Autodesk Fusion 360 part; units mm, degrees
(part 2 of 5)
sketch "Sketch20" plane through (0, 0, 3.3) normal (0, 0, 1) x (-1, 0, 0)
  arc A0 (-66.5616, 3.5945) -> (-66.8099, 2.6679) centre (-55, 0) ccw
  arc A1 (-67.9306, 1.8988) -> (-66.8099, 2.6679) centre (-67.7853, 2.8882) ccw
  line L0 (-67.9306, 1.8988) -> (-68.9458, 2.0479)
  spline S0 degree 5 poles (-68.9458, 2.0479) (-68.9559, 2.0494) (-68.9759, 2.052) (-69.0061, 2.055) (-69.0465, 2.0571) (-69.0972, 2.0572) (-69.1481, 2.0556) (-69.199, 2.0528) (-69.2501, 2.0495) (-69.3011, 2.0457) (-69.3522, 2.0415) (-69.4034, 2.0367) (-69.4546, 2.0311) (-69.5058, 2.0247) (-69.5571, 2.0173) (-69.6084, 2.0092) (-69.6597, 2.0003) (-69.7111, 1.9908) (-69.7624, 1.9808) (-69.8137, 1.9703) (-69.8651, 1.9594) (-69.9164, 1.9479) (-69.9678, 1.9358) (-70.0191, 1.9232) (-70.0705, 1.91) (-70.1218, 1.8963) (-70.1731, 1.882) (-70.2244, 1.8673) (-70.2757, 1.8521) (-70.3269, 1.8365) (-70.3781, 1.8204) (-70.4293, 1.8038) (-70.4805, 1.7868) (-70.5316, 1.7693) (-70.5827, 1.7513) (-70.6338, 1.7329) (-70.6848, 1.7141) (-70.7358, 1.6948) (-70.7868, 1.6751) (-70.8377, 1.655) (-70.8886, 1.6345) (-70.9394, 1.6136) (-70.9902, 1.5922) (-71.0409, 1.5705) (-71.0916, 1.5483) (-71.1422, 1.5258) (-71.1928, 1.5028) (-71.2433, 1.4794) (-71.2937, 1.4557) (-71.3441, 1.4316) (-71.3944, 1.4071) (-71.4447, 1.3822) (-71.4949, 1.3569) (-71.545, 1.3313) (-71.5951, 1.3053) (-71.6451, 1.2789) (-71.695, 1.2521) (-71.7448, 1.225) (-71.7946, 1.1975) (-71.8443, 1.1697) (-71.8939, 1.1415) (-71.9435, 1.1129) (-71.9929, 1.084) (-72.0423, 1.0548) (-72.0916, 1.0251) (-72.1408, 0.9952) (-72.1899, 0.9649) (-72.239, 0.9343) (-72.2879, 0.9033) (-72.3368, 0.8719) (-72.3856, 0.8403) (-72.4245, 0.8147) (-72.4537, 0.7953) (-72.4731, 0.7824) (-72.4828, 0.7759) knots 0 0 0 0 0 0 0.01428571 0.02857143 0.04285714 0.05714286 0.07142857 0.08571429 0.1 0.11428571 0.12857143 0.14285714 0.15714286 0.17142857 0.18571429 0.2 0.21428571 0.22857143 0.24285714 0.25714286 0.27142857 0.28571429 0.3 0.31428571 0.32857143 0.34285714 0.35714286 0.37142857 0.38571429 0.4 0.41428571 0.42857143 0.44285714 0.45714286 0.47142857 0.48571429 0.5 0.51428571 0.52857143 0.54285714 0.55714286 0.57142857 0.58571429 0.6 0.61428571 0.62857143 0.64285714 0.65714286 0.67142857 0.68571429 0.7 0.71428571 0.72857143 0.74285714 0.75714286 0.77142857 0.78571429 0.8 0.81428571 0.82857143 0.84285714 0.85714286 0.87142857 0.88571429 0.9 0.91428571 0.92857143 0.94285714 0.95714286 0.97142857 0.98571429 1 1 1 1 1 1
  arc A2 (-72.4828, 0.7759) -> (-72.4828, -0.7759) centre (-55, 0) ccw
  spline S1 degree 5 poles (-72.4828, -0.7759) (-72.4731, -0.7824) (-72.4537, -0.7953) (-72.4245, -0.8147) (-72.3856, -0.8403) (-72.3368, -0.8719) (-72.2879, -0.9033) (-72.239, -0.9343) (-72.1899, -0.9649) (-72.1408, -0.9952) (-72.0916, -1.0251) (-72.0423, -1.0548) (-71.9929, -1.084) (-71.9435, -1.1129) (-71.8939, -1.1415) (-71.8443, -1.1697) (-71.7946, -1.1975) (-71.7448, -1.225) (-71.695, -1.2521) (-71.6451, -1.2789) (-71.5951, -1.3053) (-71.545, -1.3313) (-71.4949, -1.3569) (-71.4447, -1.3822) (-71.3944, -1.4071) (-71.3441, -1.4316) (-71.2937, -1.4557) (-71.2433, -1.4794) (-71.1928, -1.5028) (-71.1422, -1.5258) (-71.0916, -1.5483) (-71.0409, -1.5705) (-70.9902, -1.5922) (-70.9394, -1.6136) (-70.8886, -1.6345) (-70.8377, -1.655) (-70.7868, -1.6751) (-70.7358, -1.6948) (-70.6848, -1.7141) (-70.6338, -1.7329) (-70.5827, -1.7513) (-70.5316, -1.7693) (-70.4805, -1.7868) (-70.4293, -1.8038) (-70.3781, -1.8204) (-70.3269, -1.8365) (-70.2757, -1.8521) (-70.2244, -1.8673) (-70.1731, -1.882) (-70.1218, -1.8963) (-70.0705, -1.91) (-70.0191, -1.9232) (-69.9678, -1.9358) (-69.9164, -1.9479) (-69.8651, -1.9594) (-69.8137, -1.9703) (-69.7624, -1.9808) (-69.7111, -1.9908) (-69.6597, -2.0003) (-69.6084, -2.0092) (-69.5571, -2.0173) (-69.5058, -2.0247) (-69.4546, -2.0311) (-69.4034, -2.0367) (-69.3522, -2.0415) (-69.3011, -2.0457) (-69.2501, -2.0495) (-69.199, -2.0528) (-69.1481, -2.0556) (-69.0972, -2.0572) (-69.0465, -2.0571) (-69.0061, -2.055) (-68.9759, -2.052) (-68.9559, -2.0494) (-68.9458, -2.0479) knots -1 -1 -1 -1 -1 -1 -0.98571429 -0.97142857 -0.95714286 -0.94285714 -0.92857143 -0.91428571 -0.9 -0.88571429 -0.87142857 -0.85714286 -0.84285714 -0.82857143 -0.81428571 -0.8 -0.78571429 -0.77142857 -0.75714286 -0.74285714 -0.72857143 -0.71428571 -0.7 -0.68571429 -0.67142857 -0.65714286 -0.64285714 -0.62857143 -0.61428571 -0.6 -0.58571429 -0.57142857 -0.55714286 -0.54285714 -0.52857143 -0.51428571 -0.5 -0.48571429 -0.47142857 -0.45714286 -0.44285714 -0.42857143 -0.41428571 -0.4 -0.38571429 -0.37142857 -0.35714286 -0.34285714 -0.32857143 -0.31428571 -0.3 -0.28571429 -0.27142857 -0.25714286 -0.24285714 -0.22857143 -0.21428571 -0.2 -0.18571429 -0.17142857 -0.15714286 -0.14285714 -0.12857143 -0.11428571 -0.1 -0.08571429 -0.07142857 -0.05714286 -0.04285714 -0.02857143 -0.01428571 0 0 0 0 0 0
  line L1 (-68.9458, -2.0479) -> (-67.9306, -1.8988)
  arc A3 (-66.8099, -2.6679) -> (-67.9306, -1.8988) centre (-67.7853, -2.8882) ccw
  arc A4 (-66.8099, -2.6679) -> (-66.5616, -3.5945) centre (-55, 0) ccw
  arc A5 (-67.1477, -4.8209) -> (-66.5616, -3.5945) centre (-67.5165, -3.8914) ccw
  line L2 (-67.1477, -4.8209) -> (-68.1014, -5.1994)
  spline S2 degree 5 poles (-68.1014, -5.1994) (-68.1108, -5.2031) (-68.1295, -5.2109) (-68.1571, -5.2234) (-68.1932, -5.2418) (-68.2372, -5.267) (-68.2804, -5.2939) (-68.3231, -5.3217) (-68.3657, -5.3501) (-68.408, -5.3789) (-68.4502, -5.4081) (-68.4921, -5.4379) (-68.5336, -5.4683) (-68.5747, -5.4995) (-68.6155, -5.5315) (-68.6558, -5.5642) (-68.6958, -5.5976) (-68.7355, -5.6314) (-68.775, -5.6658) (-68.8143, -5.7005) (-68.8532, -5.7357) (-68.8919, -5.7713) (-68.9304, -5.8074) (-68.9685, -5.844) (-69.0064, -5.8811) (-69.044, -5.9187) (-69.0813, -5.9566) (-69.1184, -5.995) (-69.1552, -6.0338) (-69.1917, -6.073) (-69.228, -6.1126) (-69.2641, -6.1525) (-69.2999, -6.1929) (-69.3354, -6.2336) (-69.3707, -6.2747) (-69.4057, -6.3161) (-69.4405, -6.358) (-69.4751, -6.4002) (-69.5093, -6.4427) (-69.5434, -6.4856) (-69.5772, -6.5288) (-69.6107, -6.5723) (-69.644, -6.6162) (-69.6771, -6.6604) (-69.7099, -6.7049) (-69.7424, -6.7498) (-69.7747, -6.7949) (-69.8068, -6.8404) (-69.8386, -6.8862) (-69.8702, -6.9323) (-69.9015, -6.9787) (-69.9326, -7.0253) (-69.9634, -7.0723) (-69.994, -7.1196) (-70.0244, -7.1672) (-70.0545, -7.215) (-70.0843, -7.2631) (-70.114, -7.3115) (-70.1433, -7.3602) (-70.1724, -7.4092) (-70.2013, -7.4584) (-70.2299, -7.5079) (-70.2583, -7.5577) (-70.2865, -7.6077) (-70.3143, -7.658) (-70.342, -7.7085) (-70.3694, -7.7594) (-70.3965, -7.8104) (-70.4234, -7.8617) (-70.4501, -7.9133) (-70.4765, -7.9651) (-70.4974, -8.0067) (-70.513, -8.038) (-70.5233, -8.059) (-70.5285, -8.0695) knots 0 0 0 0 0 0 0.01428571 0.02857143 0.04285714 0.05714286 0.07142857 0.08571429 0.1 0.11428571 0.12857143 0.14285714 0.15714286 0.17142857 0.18571429 0.2 0.21428571 0.22857143 0.24285714 0.25714286 0.27142857 0.28571429 0.3 0.31428571 0.32857143 0.34285714 0.35714286 0.37142857 0.38571429 0.4 0.41428571 0.42857143 0.44285714 0.45714286 0.47142857 0.48571429 0.5 0.51428571 0.52857143 0.54285714 0.55714286 0.57142857 0.58571429 0.6 0.61428571 0.62857143 0.64285714 0.65714286 0.67142857 0.68571429 0.7 0.71428571 0.72857143 0.74285714 0.75714286 0.77142857 0.78571429 0.8 0.81428571 0.82857143 0.84285714 0.85714286 0.87142857 0.88571429 0.9 0.91428571 0.92857143 0.94285714 0.95714286 0.97142857 0.98571429 1 1 1 1 1 1
  arc A6 (-70.5285, -8.0695) -> (-69.7526, -9.4133) centre (-55, 0) ccw
  spline S3 degree 5 poles (-69.7526, -9.4133) (-69.741, -9.4141) (-69.7176, -9.4156) (-69.6827, -9.4178) (-69.6362, -9.4205) (-69.5781, -9.4235) (-69.5202, -9.4262) (-69.4623, -9.4286) (-69.4045, -9.4306) (-69.3468, -9.4323) (-69.2892, -9.4336) (-69.2317, -9.4346) (-69.1743, -9.4353) (-69.117, -9.4356) (-69.0598, -9.4355) (-69.0028, -9.4351) (-68.9458, -9.4344) (-68.889, -9.4333) (-68.8322, -9.4319) (-68.7756, -9.4301) (-68.7191, -9.4279) (-68.6628, -9.4254) (-68.6065, -9.4226) (-68.5504, -9.4193) (-68.4945, -9.4158) (-68.4386, -9.4118) (-68.3829, -9.4075) (-68.3274, -9.4029) (-68.2719, -9.3978) (-68.2167, -9.3924) (-68.1616, -9.3867) (-68.1066, -9.3805) (-68.0518, -9.374) (-67.9971, -9.3671) (-67.9427, -9.3598) (-67.8883, -9.3522) (-67.8342, -9.3441) (-67.7802, -9.3357) (-67.7264, -9.3269) (-67.6728, -9.3177) (-67.6194, -9.3081) (-67.5662, -9.298) (-67.5131, -9.2876) (-67.4603, -9.2768) (-67.4077, -9.2655) (-67.3552, -9.2539) (-67.303, -9.2418) (-67.251, -9.2293) (-67.1993, -9.2164) (-67.1477, -9.2031) (-67.0964, -9.1893) (-67.0454, -9.1751) (-66.9946, -9.1603) (-66.9441, -9.1451) (-66.8939, -9.1294) (-66.8439, -9.1132) (-66.7942, -9.0966) (-66.7447, -9.0796) (-66.6955, -9.0621) (-66.6467, -9.0442) (-66.5981, -9.0256) (-66.5501, -9.0063) (-66.5025, -8.9863) (-66.4554, -8.9655) (-66.4087, -8.9441) (-66.3623, -8.9222) (-66.3162, -8.8999) (-66.2703, -8.8773) (-66.2248, -8.8542) (-66.1799, -8.8302) (-66.1361, -8.8047) (-66.1022, -8.7827) (-66.0775, -8.765) (-66.0614, -8.7527) (-66.0535, -8.7464) knots -1 -1 -1 -1 -1 -1 -0.98571429 -0.97142857 -0.95714286 -0.94285714 -0.92857143 -0.91428571 -0.9 -0.88571429 -0.87142857 -0.85714286 -0.84285714 -0.82857143 -0.81428571 -0.8 -0.78571429 -0.77142857 -0.75714286 -0.74285714 -0.72857143 -0.71428571 -0.7 -0.68571429 -0.67142857 -0.65714286 -0.64285714 -0.62857143 -0.61428571 -0.6 -0.58571429 -0.57142857 -0.55714286 -0.54285714 -0.52857143 -0.51428571 -0.5 -0.48571429 -0.47142857 -0.45714286 -0.44285714 -0.42857143 -0.41428571 -0.4 -0.38571429 -0.37142857 -0.35714286 -0.34285714 -0.32857143 -0.31428571 -0.3 -0.28571429 -0.27142857 -0.25714286 -0.24285714 -0.22857143 -0.21428571 -0.2 -0.18571429 -0.17142857 -0.15714286 -0.14285714 -0.12857143 -0.11428571 -0.1 -0.08571429 -0.07142857 -0.05714286 -0.04285714 -0.02857143 -0.01428571 0 0 0 0 0 0
  line L3 (-66.0535, -8.7464) -> (-65.2488, -8.1097)
  arc A7 (-63.8938, -8.2154) -> (-65.2488, -8.1097) centre (-64.6283, -8.8939) ccw
  arc A8 (-63.8938, -8.2154) -> (-63.2154, -8.8938) centre (-55, 0) ccw
  arc A9 (-63.1097, -10.2488) -> (-63.2154, -8.8938) centre (-63.8939, -9.6283) ccw
  line L4 (-63.1097, -10.2488) -> (-63.7464, -11.0535)
  spline S4 degree 5 poles (-63.7464, -11.0535) (-63.7527, -11.0614) (-63.765, -11.0775) (-63.7827, -11.1022) (-63.8047, -11.1361) (-63.8302, -11.1799) (-63.8542, -11.2248) (-63.8773, -11.2703) (-63.8999, -11.3162) (-63.9222, -11.3623) (-63.9441, -11.4087) (-63.9655, -11.4554) (-63.9863, -11.5025) (-64.0063, -11.5501) (-64.0256, -11.5981) (-64.0442, -11.6467) (-64.0621, -11.6955) (-64.0796, -11.7447) (-64.0966, -11.7942) (-64.1132, -11.8439) (-64.1294, -11.8939) (-64.1451, -11.9441) (-64.1603, -11.9946) (-64.1751, -12.0454) (-64.1893, -12.0964) (-64.2031, -12.1477) (-64.2164, -12.1993) (-64.2293, -12.251) (-64.2418, -12.303) (-64.2539, -12.3552) (-64.2655, -12.4077) (-64.2768, -12.4603) (-64.2876, -12.5131) (-64.298, -12.5662) (-64.3081, -12.6194) (-64.3177, -12.6728) (-64.3269, -12.7264) (-64.3357, -12.7802) (-64.3441, -12.8342) (-64.3522, -12.8883) (-64.3598, -12.9427) (-64.3671, -12.9971) (-64.374, -13.0518) (-64.3805, -13.1066) (-64.3867, -13.1616) (-64.3924, -13.2167) (-64.3978, -13.2719) (-64.4029, -13.3274) (-64.4075, -13.3829) (-64.4118, -13.4386) (-64.4158, -13.4945) (-64.4193, -13.5504) (-64.4226, -13.6065) (-64.4254, -13.6628) (-64.4279, -13.7191) (-64.4301, -13.7756) (-64.4319, -13.8322) (-64.4333, -13.889) (-64.4344, -13.9458) (-64.4351, -14.0028) (-64.4355, -14.0598) (-64.4356, -14.117) (-64.4353, -14.1743) (-64.4346, -14.2317) (-64.4336, -14.2892) (-64.4323, -14.3468) (-64.4306, -14.4045) (-64.4286, -14.4623) (-64.4262, -14.5202) (-64.4235, -14.5781) (-64.4205, -14.6362) (-64.4178, -14.6827) (-64.4156, -14.7176) (-64.4141, -14.741) (-64.4133, -14.7526) knots 0 0 0 0 0 0 0.01428571 0.02857143 0.04285714 0.05714286 0.07142857 0.08571429 0.1 0.11428571 0.12857143 0.14285714 0.15714286 0.17142857 0.18571429 0.2 0.21428571 0.22857143 0.24285714 0.25714286 0.27142857 0.28571429 0.3 0.31428571 0.32857143 0.34285714 0.35714286 0.37142857 0.38571429 0.4 0.41428571 0.42857143 0.44285714 0.45714286 0.47142857 0.48571429 0.5 0.51428571 0.52857143 0.54285714 0.55714286 0.57142857 0.58571429 0.6 0.61428571 0.62857143 0.64285714 0.65714286 0.67142857 0.68571429 0.7 0.71428571 0.72857143 0.74285714 0.75714286 0.77142857 0.78571429 0.8 0.81428571 0.82857143 0.84285714 0.85714286 0.87142857 0.88571429 0.9 0.91428571 0.92857143 0.94285714 0.95714286 0.97142857 0.98571429 1 1 1 1 1 1
  arc A10 (-64.4133, -14.7526) -> (-63.0695, -15.5285) centre (-55, 0) ccw
  spline S5 degree 5 poles (-63.0695, -15.5285) (-63.059, -15.5233) (-63.038, -15.513) (-63.0067, -15.4974) (-62.9651, -15.4765) (-62.9133, -15.4501) (-62.8617, -15.4234) (-62.8104, -15.3965) (-62.7594, -15.3694) (-62.7085, -15.342) (-62.658, -15.3143) (-62.6077, -15.2865) (-62.5577, -15.2583) (-62.5079, -15.2299) (-62.4584, -15.2013) (-62.4092, -15.1724) (-62.3602, -15.1433) (-62.3115, -15.114) (-62.2631, -15.0843) (-62.215, -15.0545) (-62.1672, -15.0244) (-62.1196, -14.994) (-62.0723, -14.9634) (-62.0253, -14.9326) (-61.9787, -14.9015) (-61.9323, -14.8702) (-61.8862, -14.8386) (-61.8404, -14.8068) (-61.7949, -14.7747) (-61.7498, -14.7424) (-61.7049, -14.7099) (-61.6604, -14.6771) (-61.6162, -14.644) (-61.5723, -14.6107) (-61.5288, -14.5772) (-61.4856, -14.5434) (-61.4427, -14.5093) (-61.4002, -14.4751) (-61.358, -14.4405) (-61.3161, -14.4057) (-61.2747, -14.3707) (-61.2336, -14.3354) (-61.1929, -14.2999) (-61.1525, -14.2641) (-61.1126, -14.228) (-61.073, -14.1917) (-61.0338, -14.1552) (-60.995, -14.1184) (-60.9566, -14.0813) (-60.9187, -14.044) (-60.8811, -14.0064) (-60.844, -13.9685) (-60.8074, -13.9304) (-60.7713, -13.8919) (-60.7357, -13.8532) (-60.7005, -13.8143) (-60.6658, -13.775) (-60.6314, -13.7355) (-60.5976, -13.6958) (-60.5642, -13.6558) (-60.5315, -13.6155) (-60.4995, -13.5747) (-60.4683, -13.5336) (-60.4379, -13.4921) (-60.4081, -13.4502) (-60.3789, -13.408) (-60.3501, -13.3657) (-60.3217, -13.3231) (-60.2939, -13.2804) (-60.267, -13.2372) (-60.2418, -13.1932) (-60.2234, -13.1571) (-60.2109, -13.1295) (-60.2031, -13.1108) (-60.1994, -13.1014) knots -1 -1 -1 -1 -1 -1 -0.98571429 -0.97142857 -0.95714286 -0.94285714 -0.92857143 -0.91428571 -0.9 -0.88571429 -0.87142857 -0.85714286 -0.84285714 -0.82857143 -0.81428571 -0.8 -0.78571429 -0.77142857 -0.75714286 -0.74285714 -0.72857143 -0.71428571 -0.7 -0.68571429 -0.67142857 -0.65714286 -0.64285714 -0.62857143 -0.61428571 -0.6 -0.58571429 -0.57142857 -0.55714286 -0.54285714 -0.52857143 -0.51428571 -0.5 -0.48571429 -0.47142857 -0.45714286 -0.44285714 -0.42857143 -0.41428571 -0.4 -0.38571429 -0.37142857 -0.35714286 -0.34285714 -0.32857143 -0.31428571 -0.3 -0.28571429 -0.27142857 -0.25714286 -0.24285714 -0.22857143 -0.21428571 -0.2 -0.18571429 -0.17142857 -0.15714286 -0.14285714 -0.12857143 -0.11428571 -0.1 -0.08571429 -0.07142857 -0.05714286 -0.04285714 -0.02857143 -0.01428571 0 0 0 0 0 0
  line L5 (-60.1994, -13.1014) -> (-59.8209, -12.1477)
  arc A11 (-58.5945, -11.5616) -> (-59.8209, -12.1477) centre (-58.8914, -12.5165) ccw
  arc A12 (-58.5945, -11.5616) -> (-57.6679, -11.8099) centre (-55, 0) ccw
  arc A13 (-56.8988, -12.9306) -> (-57.6679, -11.8099) centre (-57.8882, -12.7853) ccw
  line L6 (-56.8988, -12.9306) -> (-57.0479, -13.9458)
  spline S6 degree 5 poles (-57.0479, -13.9458) (-57.0494, -13.9559) (-57.052, -13.9759) (-57.055, -14.0061) (-57.0571, -14.0465) (-57.0572, -14.0972) (-57.0556, -14.1481) (-57.0528, -14.199) (-57.0495, -14.2501) (-57.0457, -14.3011) (-57.0415, -14.3522) (-57.0367, -14.4034) (-57.0311, -14.4546) (-57.0247, -14.5058) (-57.0173, -14.5571) (-57.0092, -14.6084) (-57.0003, -14.6597) (-56.9908, -14.7111) (-56.9808, -14.7624) (-56.9703, -14.8137) (-56.9594, -14.8651) (-56.9479, -14.9164) (-56.9358, -14.9678) (-56.9232, -15.0191) (-56.91, -15.0705) (-56.8963, -15.1218) (-56.882, -15.1731) (-56.8673, -15.2244) (-56.8521, -15.2757) (-56.8365, -15.3269) (-56.8204, -15.3781) (-56.8038, -15.4293) (-56.7868, -15.4805) (-56.7693, -15.5316) (-56.7513, -15.5827) (-56.7329, -15.6338) (-56.7141, -15.6848) (-56.6948, -15.7358) (-56.6751, -15.7868) (-56.655, -15.8377) (-56.6345, -15.8886) (-56.6136, -15.9394) (-56.5922, -15.9902) (-56.5705, -16.0409) (-56.5483, -16.0916) (-56.5258, -16.1422) (-56.5028, -16.1928) (-56.4794, -16.2433) (-56.4557, -16.2937) (-56.4316, -16.3441) (-56.4071, -16.3944) (-56.3822, -16.4447) (-56.3569, -16.4949) (-56.3313, -16.545) (-56.3053, -16.5951) (-56.2789, -16.6451) (-56.2521, -16.695) (-56.225, -16.7448) (-56.1975, -16.7946) (-56.1697, -16.8443) (-56.1415, -16.8939) (-56.1129, -16.9435) (-56.084, -16.9929) (-56.0548, -17.0423) (-56.0251, -17.0916) (-55.9952, -17.1408) (-55.9649, -17.1899) (-55.9343, -17.239) (-55.9033, -17.2879) (-55.8719, -17.3368) (-55.8403, -17.3856) (-55.8147, -17.4245) (-55.7953, -17.4537) (-55.7824, -17.4731) (-55.7759, -17.4828) knots 0 0 0 0 0 0 0.01428571 0.02857143 0.04285714 0.05714286 0.07142857 0.08571429 0.1 0.11428571 0.12857143 0.14285714 0.15714286 0.17142857 0.18571429 0.2 0.21428571 0.22857143 0.24285714 0.25714286 0.27142857 0.28571429 0.3 0.31428571 0.32857143 0.34285714 0.35714286 0.37142857 0.38571429 0.4 0.41428571 0.42857143 0.44285714 0.45714286 0.47142857 0.48571429 0.5 0.51428571 0.52857143 0.54285714 0.55714286 0.57142857 0.58571429 0.6 0.61428571 0.62857143 0.64285714 0.65714286 0.67142857 0.68571429 0.7 0.71428571 0.72857143 0.74285714 0.75714286 0.77142857 0.78571429 0.8 0.81428571 0.82857143 0.84285714 0.85714286 0.87142857 0.88571429 0.9 0.91428571 0.92857143 0.94285714 0.95714286 0.97142857 0.98571429 1 1 1 1 1 1
  arc A14 (-55.7759, -17.4828) -> (-54.2241, -17.4828) centre (-55, 0) ccw
  spline S7 degree 5 poles (-54.2241, -17.4828) (-54.2176, -17.4731) (-54.2047, -17.4537) (-54.1853, -17.4245) (-54.1597, -17.3856) (-54.1281, -17.3368) (-54.0967, -17.2879) (-54.0657, -17.239) (-54.0351, -17.1899) (-54.0048, -17.1408) (-53.9749, -17.0916) (-53.9452, -17.0423) (-53.916, -16.9929) (-53.8871, -16.9435) (-53.8585, -16.8939) (-53.8303, -16.8443) (-53.8025, -16.7946) (-53.775, -16.7448) (-53.7479, -16.695) (-53.7211, -16.6451) (-53.6947, -16.5951) (-53.6687, -16.545) (-53.6431, -16.4949) (-53.6178, -16.4447) (-53.5929, -16.3944) (-53.5684, -16.3441) (-53.5443, -16.2937) (-53.5206, -16.2433) (-53.4972, -16.1928) (-53.4742, -16.1422) (-53.4517, -16.0916) (-53.4295, -16.0409) (-53.4078, -15.9902) (-53.3864, -15.9394) (-53.3655, -15.8886) (-53.345, -15.8377) (-53.3249, -15.7868) (-53.3052, -15.7358) (-53.2859, -15.6848) (-53.2671, -15.6338) (-53.2487, -15.5827) (-53.2307, -15.5316) (-53.2132, -15.4805) (-53.1962, -15.4293) (-53.1796, -15.3781) (-53.1635, -15.3269) (-53.1479, -15.2757) (-53.1327, -15.2244) (-53.118, -15.1731) (-53.1037, -15.1218) (-53.09, -15.0705) (-53.0768, -15.0191) (-53.0642, -14.9678) (-53.0521, -14.9164) (-53.0406, -14.8651) (-53.0297, -14.8137) (-53.0192, -14.7624) (-53.0092, -14.7111) (-52.9997, -14.6597) (-52.9908, -14.6084) (-52.9827, -14.5571) (-52.9753, -14.5058) (-52.9689, -14.4546) (-52.9633, -14.4034) (-52.9585, -14.3522) (-52.9543, -14.3011) (-52.9505, -14.2501) (-52.9472, -14.199) (-52.9444, -14.1481) (-52.9428, -14.0972) (-52.9429, -14.0465) (-52.945, -14.0061) (-52.948, -13.9759) (-52.9506, -13.9559) (-52.9521, -13.9458) knots -1 -1 -1 -1 -1 -1 -0.98571429 -0.97142857 -0.95714286 -0.94285714 -0.92857143 -0.91428571 -0.9 -0.88571429 -0.87142857 -0.85714286 -0.84285714 -0.82857143 -0.81428571 -0.8 -0.78571429 -0.77142857 -0.75714286 -0.74285714 -0.72857143 -0.71428571 -0.7 -0.68571429 -0.67142857 -0.65714286 -0.64285714 -0.62857143 -0.61428571 -0.6 -0.58571429 -0.57142857 -0.55714286 -0.54285714 -0.52857143 -0.51428571 -0.5 -0.48571429 -0.47142857 -0.45714286 -0.44285714 -0.42857143 -0.41428571 -0.4 -0.38571429 -0.37142857 -0.35714286 -0.34285714 -0.32857143 -0.31428571 -0.3 -0.28571429 -0.27142857 -0.25714286 -0.24285714 -0.22857143 -0.21428571 -0.2 -0.18571429 -0.17142857 -0.15714286 -0.14285714 -0.12857143 -0.11428571 -0.1 -0.08571429 -0.07142857 -0.05714286 -0.04285714 -0.02857143 -0.01428571 0 0 0 0 0 0
  line L7 (-52.9521, -13.9458) -> (-53.1012, -12.9306)
  arc A15 (-52.3321, -11.8099) -> (-53.1012, -12.9306) centre (-52.1118, -12.7853) ccw
  arc A16 (-52.3321, -11.8099) -> (-51.4055, -11.5616) centre (-55, 0) ccw
  arc A17 (-50.1791, -12.1477) -> (-51.4055, -11.5616) centre (-51.1086, -12.5165) ccw
  line L8 (-50.1791, -12.1477) -> (-49.8006, -13.1014)
  spline S8 degree 5 poles (-49.8006, -13.1014) (-49.7969, -13.1108) (-49.7891, -13.1295) (-49.7766, -13.1571) (-49.7582, -13.1932) (-49.733, -13.2372) (-49.7061, -13.2804) (-49.6783, -13.3231) (-49.6499, -13.3657) (-49.6211, -13.408) (-49.5919, -13.4502) (-49.5621, -13.4921) (-49.5317, -13.5336) (-49.5005, -13.5747) (-49.4685, -13.6155) (-49.4358, -13.6558) (-49.4024, -13.6958) (-49.3686, -13.7355) (-49.3342, -13.775) (-49.2995, -13.8143) (-49.2643, -13.8532) (-49.2287, -13.8919) (-49.1926, -13.9304) (-49.156, -13.9685) (-49.1189, -14.0064) (-49.0813, -14.044) (-49.0434, -14.0813) (-49.005, -14.1184) (-48.9662, -14.1552) (-48.927, -14.1917) (-48.8874, -14.228) (-48.8475, -14.2641) (-48.8071, -14.2999) (-48.7664, -14.3354) (-48.7253, -14.3707) (-48.6839, -14.4057) (-48.642, -14.4405) (-48.5998, -14.4751) (-48.5573, -14.5093) (-48.5144, -14.5434) (-48.4712, -14.5772) (-48.4277, -14.6107) (-48.3838, -14.644) (-48.3396, -14.6771) (-48.2951, -14.7099) (-48.2502, -14.7424) (-48.2051, -14.7747) (-48.1596, -14.8068) (-48.1138, -14.8386) (-48.0677, -14.8702) (-48.0213, -14.9015) (-47.9747, -14.9326) (-47.9277, -14.9634) (-47.8804, -14.994) (-47.8328, -15.0244) (-47.785, -15.0545) (-47.7369, -15.0843) (-47.6885, -15.114) (-47.6398, -15.1433) (-47.5908, -15.1724) (-47.5416, -15.2013) (-47.4921, -15.2299) (-47.4423, -15.2583) (-47.3923, -15.2865) (-47.342, -15.3143) (-47.2915, -15.342) (-47.2406, -15.3694) (-47.1896, -15.3965) (-47.1383, -15.4234) (-47.0867, -15.4501) (-47.0349, -15.4765) (-46.9933, -15.4974) (-46.962, -15.513) (-46.941, -15.5233) (-46.9305, -15.5285) knots 0 0 0 0 0 0 0.01428571 0.02857143 0.04285714 0.05714286 0.07142857 0.08571429 0.1 0.11428571 0.12857143 0.14285714 0.15714286 0.17142857 0.18571429 0.2 0.21428571 0.22857143 0.24285714 0.25714286 0.27142857 0.28571429 0.3 0.31428571 0.32857143 0.34285714 0.35714286 0.37142857 0.38571429 0.4 0.41428571 0.42857143 0.44285714 0.45714286 0.47142857 0.48571429 0.5 0.51428571 0.52857143 0.54285714 0.55714286 0.57142857 0.58571429 0.6 0.61428571 0.62857143 0.64285714 0.65714286 0.67142857 0.68571429 0.7 0.71428571 0.72857143 0.74285714 0.75714286 0.77142857 0.78571429 0.8 0.81428571 0.82857143 0.84285714 0.85714286 0.87142857 0.88571429 0.9 0.91428571 0.92857143 0.94285714 0.95714286 0.97142857 0.98571429 1 1 1 1 1 1
  arc A18 (-46.9305, -15.5285) -> (-45.5867, -14.7526) centre (-55, 0) ccw
  spline S9 degree 5 poles (-45.5867, -14.7526) (-45.5859, -14.741) (-45.5844, -14.7176) (-45.5822, -14.6827) (-45.5795, -14.6362) (-45.5765, -14.5781) (-45.5738, -14.5202) (-45.5714, -14.4623) (-45.5694, -14.4045) (-45.5677, -14.3468) (-45.5664, -14.2892) (-45.5654, -14.2317) (-45.5647, -14.1743) (-45.5644, -14.117) (-45.5645, -14.0598) (-45.5649, -14.0028) (-45.5656, -13.9458) (-45.5667, -13.889) (-45.5681, -13.8322) (-45.5699, -13.7756) (-45.5721, -13.7191) (-45.5746, -13.6628) (-45.5774, -13.6065) (-45.5807, -13.5504) (-45.5842, -13.4945) (-45.5882, -13.4386) (-45.5925, -13.3829) (-45.5971, -13.3274) (-45.6022, -13.2719) (-45.6076, -13.2167) (-45.6133, -13.1616) (-45.6195, -13.1066) (-45.626, -13.0518) (-45.6329, -12.9971) (-45.6402, -12.9427) (-45.6478, -12.8883) (-45.6559, -12.8342) (-45.6643, -12.7802) (-45.6731, -12.7264) (-45.6823, -12.6728) (-45.6919, -12.6194) (-45.702, -12.5662) (-45.7124, -12.5131) (-45.7232, -12.4603) (-45.7345, -12.4077) (-45.7461, -12.3552) (-45.7582, -12.303) (-45.7707, -12.251) (-45.7836, -12.1993) (-45.7969, -12.1477) (-45.8107, -12.0964) (-45.8249, -12.0454) (-45.8397, -11.9946) (-45.8549, -11.9441) (-45.8706, -11.8939) (-45.8868, -11.8439) (-45.9034, -11.7942) (-45.9204, -11.7447) (-45.9379, -11.6955) (-45.9558, -11.6467) (-45.9744, -11.5981) (-45.9937, -11.5501) (-46.0137, -11.5025) (-46.0345, -11.4554) (-46.0559, -11.4087) (-46.0778, -11.3623) (-46.1001, -11.3162) (-46.1227, -11.2703) (-46.1458, -11.2248) (-46.1698, -11.1799) (-46.1953, -11.1361) (-46.2173, -11.1022) (-46.235, -11.0775) (-46.2473, -11.0614) (-46.2536, -11.0535) knots -1 -1 -1 -1 -1 -1 -0.98571429 -0.97142857 -0.95714286 -0.94285714 -0.92857143 -0.91428571 -0.9 -0.88571429 -0.87142857 -0.85714286 -0.84285714 -0.82857143 -0.81428571 -0.8 -0.78571429 -0.77142857 -0.75714286 -0.74285714 -0.72857143 -0.71428571 -0.7 -0.68571429 -0.67142857 -0.65714286 -0.64285714 -0.62857143 -0.61428571 -0.6 -0.58571429 -0.57142857 -0.55714286 -0.54285714 -0.52857143 -0.51428571 -0.5 -0.48571429 -0.47142857 -0.45714286 -0.44285714 -0.42857143 -0.41428571 -0.4 -0.38571429 -0.37142857 -0.35714286 -0.34285714 -0.32857143 -0.31428571 -0.3 -0.28571429 -0.27142857 -0.25714286 -0.24285714 -0.22857143 -0.21428571 -0.2 -0.18571429 -0.17142857 -0.15714286 -0.14285714 -0.12857143 -0.11428571 -0.1 -0.08571429 -0.07142857 -0.05714286 -0.04285714 -0.02857143 -0.01428571 0 0 0 0 0 0
  line L9 (-46.2536, -11.0535) -> (-46.8903, -10.2488)
  arc A19 (-46.7846, -8.8938) -> (-46.8903, -10.2488) centre (-46.1061, -9.6283) ccw
  arc A20 (-46.7846, -8.8938) -> (-46.1062, -8.2154) centre (-55, 0) ccw
  arc A21 (-44.7512, -8.1097) -> (-46.1062, -8.2154) centre (-45.3717, -8.8939) ccw
  line L10 (-44.7512, -8.1097) -> (-43.9465, -8.7464)
  spline S10 degree 5 poles (-43.9465, -8.7464) (-43.9386, -8.7527) (-43.9225, -8.765) (-43.8978, -8.7827) (-43.8639, -8.8047) (-43.8201, -8.8302) (-43.7752, -8.8542) (-43.7297, -8.8773) (-43.6838, -8.8999) (-43.6377, -8.9222) (-43.5913, -8.9441) (-43.5446, -8.9655) (-43.4975, -8.9863) (-43.4499, -9.0063) (-43.4019, -9.0256) (-43.3533, -9.0442) (-43.3045, -9.0621) (-43.2553, -9.0796) (-43.2058, -9.0966) (-43.1561, -9.1132) (-43.1061, -9.1294) (-43.0559, -9.1451) (-43.0054, -9.1603) (-42.9546, -9.1751) (-42.9036, -9.1893) (-42.8523, -9.2031) (-42.8007, -9.2164) (-42.749, -9.2293) (-42.697, -9.2418) (-42.6448, -9.2539) (-42.5923, -9.2655) (-42.5397, -9.2768) (-42.4869, -9.2876) (-42.4338, -9.298) (-42.3806, -9.3081) (-42.3272, -9.3177) (-42.2736, -9.3269) (-42.2198, -9.3357) (-42.1658, -9.3441) (-42.1117, -9.3522) (-42.0573, -9.3598) (-42.0029, -9.3671) (-41.9482, -9.374) (-41.8934, -9.3805) (-41.8384, -9.3867) (-41.7833, -9.3924) (-41.7281, -9.3978) (-41.6726, -9.4029) (-41.6171, -9.4075) (-41.5614, -9.4118) (-41.5055, -9.4158) (-41.4496, -9.4193) (-41.3935, -9.4226) (-41.3372, -9.4254) (-41.2809, -9.4279) (-41.2244, -9.4301) (-41.1678, -9.4319) (-41.111, -9.4333) (-41.0542, -9.4344) (-40.9972, -9.4351) (-40.9402, -9.4355) (-40.883, -9.4356) (-40.8257, -9.4353) (-40.7683, -9.4346) (-40.7108, -9.4336) (-40.6532, -9.4323) (-40.5955, -9.4306) (-40.5377, -9.4286) (-40.4798, -9.4262) (-40.4219, -9.4235) (-40.3638, -9.4205) (-40.3173, -9.4178) (-40.2824, -9.4156) (-40.259, -9.4141) (-40.2474, -9.4133) knots 0 0 0 0 0 0 0.01428571 0.02857143 0.04285714 0.05714286 0.07142857 0.08571429 0.1 0.11428571 0.12857143 0.14285714 0.15714286 0.17142857 0.18571429 0.2 0.21428571 0.22857143 0.24285714 0.25714286 0.27142857 0.28571429 0.3 0.31428571 0.32857143 0.34285714 0.35714286 0.37142857 0.38571429 0.4 0.41428571 0.42857143 0.44285714 0.45714286 0.47142857 0.48571429 0.5 0.51428571 0.52857143 0.54285714 0.55714286 0.57142857 0.58571429 0.6 0.61428571 0.62857143 0.64285714 0.65714286 0.67142857 0.68571429 0.7 0.71428571 0.72857143 0.74285714 0.75714286 0.77142857 0.78571429 0.8 0.81428571 0.82857143 0.84285714 0.85714286 0.87142857 0.88571429 0.9 0.91428571 0.92857143 0.94285714 0.95714286 0.97142857 0.98571429 1 1 1 1 1 1
  arc A22 (-40.2474, -9.4133) -> (-39.4715, -8.0695) centre (-55, 0) ccw
  spline S11 degree 5 poles (-39.4715, -8.0695) (-39.4767, -8.059) (-39.487, -8.038) (-39.5026, -8.0067) (-39.5235, -7.9651) (-39.5499, -7.9133) (-39.5766, -7.8617) (-39.6035, -7.8104) (-39.6306, -7.7594) (-39.658, -7.7085) (-39.6857, -7.658) (-39.7135, -7.6077) (-39.7417, -7.5577) (-39.7701, -7.5079) (-39.7987, -7.4584) (-39.8276, -7.4092) (-39.8567, -7.3602) (-39.886, -7.3115) (-39.9157, -7.2631) (-39.9455, -7.215) (-39.9756, -7.1672) (-40.006, -7.1196) (-40.0366, -7.0723) (-40.0674, -7.0253) (-40.0985, -6.9787) (-40.1298, -6.9323) (-40.1614, -6.8862) (-40.1932, -6.8404) (-40.2253, -6.7949) (-40.2576, -6.7498) (-40.2901, -6.7049) (-40.3229, -6.6604) (-40.356, -6.6162) (-40.3893, -6.5723) (-40.4228, -6.5288) (-40.4566, -6.4856) (-40.4907, -6.4427) (-40.5249, -6.4002) (-40.5595, -6.358) (-40.5943, -6.3161) (-40.6293, -6.2747) (-40.6646, -6.2336) (-40.7001, -6.1929) (-40.7359, -6.1525) (-40.772, -6.1126) (-40.8083, -6.073) (-40.8448, -6.0338) (-40.8816, -5.995) (-40.9187, -5.9566) (-40.956, -5.9187) (-40.9936, -5.8811) (-41.0315, -5.844) (-41.0696, -5.8074) (-41.1081, -5.7713) (-41.1468, -5.7357) (-41.1857, -5.7005) (-41.225, -5.6658) (-41.2645, -5.6314) (-41.3042, -5.5976) (-41.3442, -5.5642) (-41.3845, -5.5315) (-41.4253, -5.4995) (-41.4664, -5.4683) (-41.5079, -5.4379) (-41.5498, -5.4081) (-41.592, -5.3789) (-41.6343, -5.3501) (-41.6769, -5.3217) (-41.7196, -5.2939) (-41.7628, -5.267) (-41.8068, -5.2418) (-41.8429, -5.2234) (-41.8705, -5.2109) (-41.8892, -5.2031) (-41.8986, -5.1994) knots -1 -1 -1 -1 -1 -1 -0.98571429 -0.97142857 -0.95714286 -0.94285714 -0.92857143 -0.91428571 -0.9 -0.88571429 -0.87142857 -0.85714286 -0.84285714 -0.82857143 -0.81428571 -0.8 -0.78571429 -0.77142857 -0.75714286 -0.74285714 -0.72857143 -0.71428571 -0.7 -0.68571429 -0.67142857 -0.65714286 -0.64285714 -0.62857143 -0.61428571 -0.6 -0.58571429 -0.57142857 -0.55714286 -0.54285714 -0.52857143 -0.51428571 -0.5 -0.48571429 -0.47142857 -0.45714286 -0.44285714 -0.42857143 -0.41428571 -0.4 -0.38571429 -0.37142857 -0.35714286 -0.34285714 -0.32857143 -0.31428571 -0.3 -0.28571429 -0.27142857 -0.25714286 -0.24285714 -0.22857143 -0.21428571 -0.2 -0.18571429 -0.17142857 -0.15714286 -0.14285714 -0.12857143 -0.11428571 -0.1 -0.08571429 -0.07142857 -0.05714286 -0.04285714 -0.02857143 -0.01428571 0 0 0 0 0 0
  line L11 (-41.8986, -5.1994) -> (-42.8523, -4.8209)
  arc A23 (-43.4384, -3.5945) -> (-42.8523, -4.8209) centre (-42.4835, -3.8914) ccw
  arc A24 (-43.4384, -3.5945) -> (-43.1901, -2.6679) centre (-55, 0) ccw
  arc A25 (-42.0694, -1.8988) -> (-43.1901, -2.6679) centre (-42.2147, -2.8882) ccw
  line L12 (-42.0694, -1.8988) -> (-41.0542, -2.0479)
  spline S12 degree 5 poles (-41.0542, -2.0479) (-41.0441, -2.0494) (-41.0241, -2.052) (-40.9939, -2.055) (-40.9535, -2.0571) (-40.9028, -2.0572) (-40.8519, -2.0556) (-40.801, -2.0528) (-40.7499, -2.0495) (-40.6989, -2.0457) (-40.6478, -2.0415) (-40.5966, -2.0367) (-40.5454, -2.0311) (-40.4942, -2.0247) (-40.4429, -2.0173) (-40.3916, -2.0092) (-40.3403, -2.0003) (-40.2889, -1.9908) (-40.2376, -1.9808) (-40.1863, -1.9703) (-40.1349, -1.9594) (-40.0836, -1.9479) (-40.0322, -1.9358) (-39.9809, -1.9232) (-39.9295, -1.91) (-39.8782, -1.8963) (-39.8269, -1.882) (-39.7756, -1.8673) (-39.7243, -1.8521) (-39.6731, -1.8365) (-39.6219, -1.8204) (-39.5707, -1.8038) (-39.5195, -1.7868) (-39.4684, -1.7693) (-39.4173, -1.7513) (-39.3662, -1.7329) (-39.3152, -1.7141) (-39.2642, -1.6948) (-39.2132, -1.6751) (-39.1623, -1.655) (-39.1114, -1.6345) (-39.0606, -1.6136) (-39.0098, -1.5922) (-38.9591, -1.5705) (-38.9084, -1.5483) (-38.8578, -1.5258) (-38.8072, -1.5028) (-38.7567, -1.4794) (-38.7063, -1.4557) (-38.6559, -1.4316) (-38.6056, -1.4071) (-38.5553, -1.3822) (-38.5051, -1.3569) (-38.455, -1.3313) (-38.4049, -1.3053) (-38.3549, -1.2789) (-38.305, -1.2521) (-38.2552, -1.225) (-38.2054, -1.1975) (-38.1557, -1.1697) (-38.1061, -1.1415) (-38.0565, -1.1129) (-38.0071, -1.084) (-37.9577, -1.0548) (-37.9084, -1.0251) (-37.8592, -0.9952) (-37.8101, -0.9649) (-37.761, -0.9343) (-37.7121, -0.9033) (-37.6632, -0.8719) (-37.6144, -0.8403) (-37.5755, -0.8147) (-37.5463, -0.7953) (-37.5269, -0.7824) (-37.5172, -0.7759) knots 0 0 0 0 0 0 0.01428571 0.02857143 0.04285714 0.05714286 0.07142857 0.08571429 0.1 0.11428571 0.12857143 0.14285714 0.15714286 0.17142857 0.18571429 0.2 0.21428571 0.22857143 0.24285714 0.25714286 0.27142857 0.28571429 0.3 0.31428571 0.32857143 0.34285714 0.35714286 0.37142857 0.38571429 0.4 0.41428571 0.42857143 0.44285714 0.45714286 0.47142857 0.48571429 0.5 0.51428571 0.52857143 0.54285714 0.55714286 0.57142857 0.58571429 0.6 0.61428571 0.62857143 0.64285714 0.65714286 0.67142857 0.68571429 0.7 0.71428571 0.72857143 0.74285714 0.75714286 0.77142857 0.78571429 0.8 0.81428571 0.82857143 0.84285714 0.85714286 0.87142857 0.88571429 0.9 0.91428571 0.92857143 0.94285714 0.95714286 0.97142857 0.98571429 1 1 1 1 1 1
  arc A26 (-37.5172, -0.7759) -> (-37.5172, 0.7759) centre (-55, 0) ccw
  spline S13 degree 5 poles (-37.5172, 0.7759) (-37.5269, 0.7824) (-37.5463, 0.7953) (-37.5755, 0.8147) (-37.6144, 0.8403) (-37.6632, 0.8719) (-37.7121, 0.9033) (-37.761, 0.9343) (-37.8101, 0.9649) (-37.8592, 0.9952) (-37.9084, 1.0251) (-37.9577, 1.0548) (-38.0071, 1.084) (-38.0565, 1.1129) (-38.1061, 1.1415) (-38.1557, 1.1697) (-38.2054, 1.1975) (-38.2552, 1.225) (-38.305, 1.2521) (-38.3549, 1.2789) (-38.4049, 1.3053) (-38.455, 1.3313) (-38.5051, 1.3569) (-38.5553, 1.3822) (-38.6056, 1.4071) (-38.6559, 1.4316) (-38.7063, 1.4557) (-38.7567, 1.4794) (-38.8072, 1.5028) (-38.8578, 1.5258) (-38.9084, 1.5483) (-38.9591, 1.5705) (-39.0098, 1.5922) (-39.0606, 1.6136) (-39.1114, 1.6345) (-39.1623, 1.655) (-39.2132, 1.6751) (-39.2642, 1.6948) (-39.3152, 1.7141) (-39.3662, 1.7329) (-39.4173, 1.7513) (-39.4684, 1.7693) (-39.5195, 1.7868) (-39.5707, 1.8038) (-39.6219, 1.8204) (-39.6731, 1.8365) (-39.7243, 1.8521) (-39.7756, 1.8673) (-39.8269, 1.882) (-39.8782, 1.8963) (-39.9295, 1.91) (-39.9809, 1.9232) (-40.0322, 1.9358) (-40.0836, 1.9479) (-40.1349, 1.9594) (-40.1863, 1.9703) (-40.2376, 1.9808) (-40.2889, 1.9908) (-40.3403, 2.0003) (-40.3916, 2.0092) (-40.4429, 2.0173) (-40.4942, 2.0247) (-40.5454, 2.0311) (-40.5966, 2.0367) (-40.6478, 2.0415) (-40.6989, 2.0457) (-40.7499, 2.0495) (-40.801, 2.0528) (-40.8519, 2.0556) (-40.9028, 2.0572) (-40.9535, 2.0571) (-40.9939, 2.055) (-41.0241, 2.052) (-41.0441, 2.0494) (-41.0542, 2.0479) knots -1 -1 -1 -1 -1 -1 -0.98571429 -0.97142857 -0.95714286 -0.94285714 -0.92857143 -0.91428571 -0.9 -0.88571429 -0.87142857 -0.85714286 -0.84285714 -0.82857143 -0.81428571 -0.8 -0.78571429 -0.77142857 -0.75714286 -0.74285714 -0.72857143 -0.71428571 -0.7 -0.68571429 -0.67142857 -0.65714286 -0.64285714 -0.62857143 -0.61428571 -0.6 -0.58571429 -0.57142857 -0.55714286 -0.54285714 -0.52857143 -0.51428571 -0.5 -0.48571429 -0.47142857 -0.45714286 -0.44285714 -0.42857143 -0.41428571 -0.4 -0.38571429 -0.37142857 -0.35714286 -0.34285714 -0.32857143 -0.31428571 -0.3 -0.28571429 -0.27142857 -0.25714286 -0.24285714 -0.22857143 -0.21428571 -0.2 -0.18571429 -0.17142857 -0.15714286 -0.14285714 -0.12857143 -0.11428571 -0.1 -0.08571429 -0.07142857 -0.05714286 -0.04285714 -0.02857143 -0.01428571 0 0 0 0 0 0
  line L13 (-41.0542, 2.0479) -> (-42.0694, 1.8988)
  arc A27 (-43.1901, 2.6679) -> (-42.0694, 1.8988) centre (-42.2147, 2.8882) ccw
  arc A28 (-43.1901, 2.6679) -> (-43.4384, 3.5945) centre (-55, 0) ccw
  arc A29 (-42.8523, 4.8209) -> (-43.4384, 3.5945) centre (-42.4835, 3.8914) ccw
  line L14 (-42.8523, 4.8209) -> (-41.8986, 5.1994)
  spline S14 degree 5 poles (-41.8986, 5.1994) (-41.8892, 5.2031) (-41.8705, 5.2109) (-41.8429, 5.2234) (-41.8068, 5.2418) (-41.7628, 5.267) (-41.7196, 5.2939) (-41.6769, 5.3217) (-41.6343, 5.3501) (-41.592, 5.3789) (-41.5498, 5.4081) (-41.5079, 5.4379) (-41.4664, 5.4683) (-41.4253, 5.4995) (-41.3845, 5.5315) (-41.3442, 5.5642) (-41.3042, 5.5976) (-41.2645, 5.6314) (-41.225, 5.6658) (-41.1857, 5.7005) (-41.1468, 5.7357) (-41.1081, 5.7713) (-41.0696, 5.8074) (-41.0315, 5.844) (-40.9936, 5.8811) (-40.956, 5.9187) (-40.9187, 5.9566) (-40.8816, 5.995) (-40.8448, 6.0338) (-40.8083, 6.073) (-40.772, 6.1126) (-40.7359, 6.1525) (-40.7001, 6.1929) (-40.6646, 6.2336) (-40.6293, 6.2747) (-40.5943, 6.3161) (-40.5595, 6.358) (-40.5249, 6.4002) (-40.4907, 6.4427) (-40.4566, 6.4856) (-40.4228, 6.5288) (-40.3893, 6.5723) (-40.356, 6.6162) (-40.3229, 6.6604) (-40.2901, 6.7049) (-40.2576, 6.7498) (-40.2253, 6.7949) (-40.1932, 6.8404) (-40.1614, 6.8862) (-40.1298, 6.9323) (-40.0985, 6.9787) (-40.0674, 7.0253) (-40.0366, 7.0723) (-40.006, 7.1196) (-39.9756, 7.1672) (-39.9455, 7.215) (-39.9157, 7.2631) (-39.886, 7.3115) (-39.8567, 7.3602) (-39.8276, 7.4092) (-39.7987, 7.4584) (-39.7701, 7.5079) (-39.7417, 7.5577) (-39.7135, 7.6077) (-39.6857, 7.658) (-39.658, 7.7085) (-39.6306, 7.7594) (-39.6035, 7.8104) (-39.5766, 7.8617) (-39.5499, 7.9133) (-39.5235, 7.9651) (-39.5026, 8.0067) (-39.487, 8.038) (-39.4767, 8.059) (-39.4715, 8.0695) knots 0 0 0 0 0 0 0.01428571 0.02857143 0.04285714 0.05714286 0.07142857 0.08571429 0.1 0.11428571 0.12857143 0.14285714 0.15714286 0.17142857 0.18571429 0.2 0.21428571 0.22857143 0.24285714 0.25714286 0.27142857 0.28571429 0.3 0.31428571 0.32857143 0.34285714 0.35714286 0.37142857 0.38571429 0.4 0.41428571 0.42857143 0.44285714 0.45714286 0.47142857 0.48571429 0.5 0.51428571 0.52857143 0.54285714 0.55714286 0.57142857 0.58571429 0.6 0.61428571 0.62857143 0.64285714 0.65714286 0.67142857 0.68571429 0.7 0.71428571 0.72857143 0.74285714 0.75714286 0.77142857 0.78571429 0.8 0.81428571 0.82857143 0.84285714 0.85714286 0.87142857 0.88571429 0.9 0.91428571 0.92857143 0.94285714 0.95714286 0.97142857 0.98571429 1 1 1 1 1 1
  arc A30 (-39.4715, 8.0695) -> (-40.2474, 9.4133) centre (-55, 0) ccw
  spline S15 degree 5 poles (-40.2474, 9.4133) (-40.259, 9.4141) (-40.2824, 9.4156) (-40.3173, 9.4178) (-40.3638, 9.4205) (-40.4219, 9.4235) (-40.4798, 9.4262) (-40.5377, 9.4286) (-40.5955, 9.4306) (-40.6532, 9.4323) (-40.7108, 9.4336) (-40.7683, 9.4346) (-40.8257, 9.4353) (-40.883, 9.4356) (-40.9402, 9.4355) (-40.9972, 9.4351) (-41.0542, 9.4344) (-41.111, 9.4333) (-41.1678, 9.4319) (-41.2244, 9.4301) (-41.2809, 9.4279) (-41.3372, 9.4254) (-41.3935, 9.4226) (-41.4496, 9.4193) (-41.5055, 9.4158) (-41.5614, 9.4118) (-41.6171, 9.4075) (-41.6726, 9.4029) (-41.7281, 9.3978) (-41.7833, 9.3924) (-41.8384, 9.3867) (-41.8934, 9.3805) (-41.9482, 9.374) (-42.0029, 9.3671) (-42.0573, 9.3598) (-42.1117, 9.3522) (-42.1658, 9.3441) (-42.2198, 9.3357) (-42.2736, 9.3269) (-42.3272, 9.3177) (-42.3806, 9.3081) (-42.4338, 9.298) (-42.4869, 9.2876) (-42.5397, 9.2768) (-42.5923, 9.2655) (-42.6448, 9.2539) (-42.697, 9.2418) (-42.749, 9.2293) (-42.8007, 9.2164) (-42.8523, 9.2031) (-42.9036, 9.1893) (-42.9546, 9.1751) (-43.0054, 9.1603) (-43.0559, 9.1451) (-43.1061, 9.1294) (-43.1561, 9.1132) (-43.2058, 9.0966) (-43.2553, 9.0796) (-43.3045, 9.0621) (-43.3533, 9.0442) (-43.4019, 9.0256) (-43.4499, 9.0063) (-43.4975, 8.9863) (-43.5446, 8.9655) (-43.5913, 8.9441) (-43.6377, 8.9222) (-43.6838, 8.8999) (-43.7297, 8.8773) (-43.7752, 8.8542) (-43.8201, 8.8302) (-43.8639, 8.8047) (-43.8978, 8.7827) (-43.9225, 8.765) (-43.9386, 8.7527) (-43.9465, 8.7464) knots -1 -1 -1 -1 -1 -1 -0.98571429 -0.97142857 -0.95714286 -0.94285714 -0.92857143 -0.91428571 -0.9 -0.88571429 -0.87142857 -0.85714286 -0.84285714 -0.82857143 -0.81428571 -0.8 -0.78571429 -0.77142857 -0.75714286 -0.74285714 -0.72857143 -0.71428571 -0.7 -0.68571429 -0.67142857 -0.65714286 -0.64285714 -0.62857143 -0.61428571 -0.6 -0.58571429 -0.57142857 -0.55714286 -0.54285714 -0.52857143 -0.51428571 -0.5 -0.48571429 -0.47142857 -0.45714286 -0.44285714 -0.42857143 -0.41428571 -0.4 -0.38571429 -0.37142857 -0.35714286 -0.34285714 -0.32857143 -0.31428571 -0.3 -0.28571429 -0.27142857 -0.25714286 -0.24285714 -0.22857143 -0.21428571 -0.2 -0.18571429 -0.17142857 -0.15714286 -0.14285714 -0.12857143 -0.11428571 -0.1 -0.08571429 -0.07142857 -0.05714286 -0.04285714 -0.02857143 -0.01428571 0 0 0 0 0 0
  line L15 (-43.9465, 8.7464) -> (-44.7512, 8.1097)
  arc A31 (-46.1062, 8.2154) -> (-44.7512, 8.1097) centre (-45.3717, 8.8939) ccw
  arc A32 (-46.1062, 8.2154) -> (-46.7846, 8.8938) centre (-55, 0) ccw
  arc A33 (-46.8903, 10.2488) -> (-46.7846, 8.8938) centre (-46.1061, 9.6283) ccw
  line L16 (-46.8903, 10.2488) -> (-46.2536, 11.0535)
  spline S16 degree 5 poles (-46.2536, 11.0535) (-46.2473, 11.0614) (-46.235, 11.0775) (-46.2173, 11.1022) (-46.1953, 11.1361) (-46.1698, 11.1799) (-46.1458, 11.2248) (-46.1227, 11.2703) (-46.1001, 11.3162) (-46.0778, 11.3623) (-46.0559, 11.4087) (-46.0345, 11.4554) (-46.0137, 11.5025) (-45.9937, 11.5501) (-45.9744, 11.5981) (-45.9558, 11.6467) (-45.9379, 11.6955) (-45.9204, 11.7447) (-45.9034, 11.7942) (-45.8868, 11.8439) (-45.8706, 11.8939) (-45.8549, 11.9441) (-45.8397, 11.9946) (-45.8249, 12.0454) (-45.8107, 12.0964) (-45.7969, 12.1477) (-45.7836, 12.1993) (-45.7707, 12.251) (-45.7582, 12.303) (-45.7461, 12.3552) (-45.7345, 12.4077) (-45.7232, 12.4603) (-45.7124, 12.5131) (-45.702, 12.5662) (-45.6919, 12.6194) (-45.6823, 12.6728) (-45.6731, 12.7264) (-45.6643, 12.7802) (-45.6559, 12.8342) (-45.6478, 12.8883) (-45.6402, 12.9427) (-45.6329, 12.9971) (-45.626, 13.0518) (-45.6195, 13.1066) (-45.6133, 13.1616) (-45.6076, 13.2167) (-45.6022, 13.2719) (-45.5971, 13.3274) (-45.5925, 13.3829) (-45.5882, 13.4386) (-45.5842, 13.4945) (-45.5807, 13.5504) (-45.5774, 13.6065) (-45.5746, 13.6628) (-45.5721, 13.7191) (-45.5699, 13.7756) (-45.5681, 13.8322) (-45.5667, 13.889) (-45.5656, 13.9458) (-45.5649, 14.0028) (-45.5645, 14.0598) (-45.5644, 14.117) (-45.5647, 14.1743) (-45.5654, 14.2317) (-45.5664, 14.2892) (-45.5677, 14.3468) (-45.5694, 14.4045) (-45.5714, 14.4623) (-45.5738, 14.5202) (-45.5765, 14.5781) (-45.5795, 14.6362) (-45.5822, 14.6827) (-45.5844, 14.7176) (-45.5859, 14.741) (-45.5867, 14.7526) knots 0 0 0 0 0 0 0.01428571 0.02857143 0.04285714 0.05714286 0.07142857 0.08571429 0.1 0.11428571 0.12857143 0.14285714 0.15714286 0.17142857 0.18571429 0.2 0.21428571 0.22857143 0.24285714 0.25714286 0.27142857 0.28571429 0.3 0.31428571 0.32857143 0.34285714 0.35714286 0.37142857 0.38571429 0.4 0.41428571 0.42857143 0.44285714 0.45714286 0.47142857 0.48571429 0.5 0.51428571 0.52857143 0.54285714 0.55714286 0.57142857 0.58571429 0.6 0.61428571 0.62857143 0.64285714 0.65714286 0.67142857 0.68571429 0.7 0.71428571 0.72857143 0.74285714 0.75714286 0.77142857 0.78571429 0.8 0.81428571 0.82857143 0.84285714 0.85714286 0.87142857 0.88571429 0.9 0.91428571 0.92857143 0.94285714 0.95714286 0.97142857 0.98571429 1 1 1 1 1 1
  arc A34 (-45.5867, 14.7526) -> (-46.9305, 15.5285) centre (-55, 0) ccw
  spline S17 degree 5 poles (-46.9305, 15.5285) (-46.941, 15.5233) (-46.962, 15.513) (-46.9933, 15.4974) (-47.0349, 15.4765) (-47.0867, 15.4501) (-47.1383, 15.4234) (-47.1896, 15.3965) (-47.2406, 15.3694) (-47.2915, 15.342) (-47.342, 15.3143) (-47.3923, 15.2865) (-47.4423, 15.2583) (-47.4921, 15.2299) (-47.5416, 15.2013) (-47.5908, 15.1724) (-47.6398, 15.1433) (-47.6885, 15.114) (-47.7369, 15.0843) (-47.785, 15.0545) (-47.8328, 15.0244) (-47.8804, 14.994) (-47.9277, 14.9634) (-47.9747, 14.9326) (-48.0213, 14.9015) (-48.0677, 14.8702) (-48.1138, 14.8386) (-48.1596, 14.8068) (-48.2051, 14.7747) (-48.2502, 14.7424) (-48.2951, 14.7099) (-48.3396, 14.6771) (-48.3838, 14.644) (-48.4277, 14.6107) (-48.4712, 14.5772) (-48.5144, 14.5434) (-48.5573, 14.5093) (-48.5998, 14.4751) (-48.642, 14.4405) (-48.6839, 14.4057) (-48.7253, 14.3707) (-48.7664, 14.3354) (-48.8071, 14.2999) (-48.8475, 14.2641) (-48.8874, 14.228) (-48.927, 14.1917) (-48.9662, 14.1552) (-49.005, 14.1184) (-49.0434, 14.0813) (-49.0813, 14.044) (-49.1189, 14.0064) (-49.156, 13.9685) (-49.1926, 13.9304) (-49.2287, 13.8919) (-49.2643, 13.8532) (-49.2995, 13.8143) (-49.3342, 13.775) (-49.3686, 13.7355) (-49.4024, 13.6958) (-49.4358, 13.6558) (-49.4685, 13.6155) (-49.5005, 13.5747) (-49.5317, 13.5336) (-49.5621, 13.4921) (-49.5919, 13.4502) (-49.6211, 13.408) (-49.6499, 13.3657) (-49.6783, 13.3231) (-49.7061, 13.2804) (-49.733, 13.2372) (-49.7582, 13.1932) (-49.7766, 13.1571) (-49.7891, 13.1295) (-49.7969, 13.1108) (-49.8006, 13.1014) knots -1 -1 -1 -1 -1 -1 -0.98571429 -0.97142857 -0.95714286 -0.94285714 -0.92857143 -0.91428571 -0.9 -0.88571429 -0.87142857 -0.85714286 -0.84285714 -0.82857143 -0.81428571 -0.8 -0.78571429 -0.77142857 -0.75714286 -0.74285714 -0.72857143 -0.71428571 -0.7 -0.68571429 -0.67142857 -0.65714286 -0.64285714 -0.62857143 -0.61428571 -0.6 -0.58571429 -0.57142857 -0.55714286 -0.54285714 -0.52857143 -0.51428571 -0.5 -0.48571429 -0.47142857 -0.45714286 -0.44285714 -0.42857143 -0.41428571 -0.4 -0.38571429 -0.37142857 -0.35714286 -0.34285714 -0.32857143 -0.31428571 -0.3 -0.28571429 -0.27142857 -0.25714286 -0.24285714 -0.22857143 -0.21428571 -0.2 -0.18571429 -0.17142857 -0.15714286 -0.14285714 -0.12857143 -0.11428571 -0.1 -0.08571429 -0.07142857 -0.05714286 -0.04285714 -0.02857143 -0.01428571 0 0 0 0 0 0
  line L17 (-49.8006, 13.1014) -> (-50.1791, 12.1477)
  arc A35 (-51.4055, 11.5616) -> (-50.1791, 12.1477) centre (-51.1086, 12.5165) ccw
  arc A36 (-51.4055, 11.5616) -> (-52.3321, 11.8099) centre (-55, 0) ccw
  arc A37 (-53.1012, 12.9306) -> (-52.3321, 11.8099) centre (-52.1118, 12.7853) ccw
  line L18 (-53.1012, 12.9306) -> (-52.9521, 13.9458)
  spline S18 degree 5 poles (-52.9521, 13.9458) (-52.9506, 13.9559) (-52.948, 13.9759) (-52.945, 14.0061) (-52.9429, 14.0465) (-52.9428, 14.0972) (-52.9444, 14.1481) (-52.9472, 14.199) (-52.9505, 14.2501) (-52.9543, 14.3011) (-52.9585, 14.3522) (-52.9633, 14.4034) (-52.9689, 14.4546) (-52.9753, 14.5058) (-52.9827, 14.5571) (-52.9908, 14.6084) (-52.9997, 14.6597) (-53.0092, 14.7111) (-53.0192, 14.7624) (-53.0297, 14.8137) (-53.0406, 14.8651) (-53.0521, 14.9164) (-53.0642, 14.9678) (-53.0768, 15.0191) (-53.09, 15.0705) (-53.1037, 15.1218) (-53.118, 15.1731) (-53.1327, 15.2244) (-53.1479, 15.2757) (-53.1635, 15.3269) (-53.1796, 15.3781) (-53.1962, 15.4293) (-53.2132, 15.4805) (-53.2307, 15.5316) (-53.2487, 15.5827) (-53.2671, 15.6338) (-53.2859, 15.6848) (-53.3052, 15.7358) (-53.3249, 15.7868) (-53.345, 15.8377) (-53.3655, 15.8886) (-53.3864, 15.9394) (-53.4078, 15.9902) (-53.4295, 16.0409) (-53.4517, 16.0916) (-53.4742, 16.1422) (-53.4972, 16.1928) (-53.5206, 16.2433) (-53.5443, 16.2937) (-53.5684, 16.3441) (-53.5929, 16.3944) (-53.6178, 16.4447) (-53.6431, 16.4949) (-53.6687, 16.545) (-53.6947, 16.5951) (-53.7211, 16.6451) (-53.7479, 16.695) (-53.775, 16.7448) (-53.8025, 16.7946) (-53.8303, 16.8443) (-53.8585, 16.8939) (-53.8871, 16.9435) (-53.916, 16.9929) (-53.9452, 17.0423) (-53.9749, 17.0916) (-54.0048, 17.1408) (-54.0351, 17.1899) (-54.0657, 17.239) (-54.0967, 17.2879) (-54.1281, 17.3368) (-54.1597, 17.3856) (-54.1853, 17.4245) (-54.2047, 17.4537) (-54.2176, 17.4731) (-54.2241, 17.4828) knots 0 0 0 0 0 0 0.01428571 0.02857143 0.04285714 0.05714286 0.07142857 0.08571429 0.1 0.11428571 0.12857143 0.14285714 0.15714286 0.17142857 0.18571429 0.2 0.21428571 0.22857143 0.24285714 0.25714286 0.27142857 0.28571429 0.3 0.31428571 0.32857143 0.34285714 0.35714286 0.37142857 0.38571429 0.4 0.41428571 0.42857143 0.44285714 0.45714286 0.47142857 0.48571429 0.5 0.51428571 0.52857143 0.54285714 0.55714286 0.57142857 0.58571429 0.6 0.61428571 0.62857143 0.64285714 0.65714286 0.67142857 0.68571429 0.7 0.71428571 0.72857143 0.74285714 0.75714286 0.77142857 0.78571429 0.8 0.81428571 0.82857143 0.84285714 0.85714286 0.87142857 0.88571429 0.9 0.91428571 0.92857143 0.94285714 0.95714286 0.97142857 0.98571429 1 1 1 1 1 1
  arc A38 (-54.2241, 17.4828) -> (-55.7759, 17.4828) centre (-55, 0) ccw
  spline S19 degree 5 poles (-55.7759, 17.4828) (-55.7824, 17.4731) (-55.7953, 17.4537) (-55.8147, 17.4245) (-55.8403, 17.3856) (-55.8719, 17.3368) (-55.9033, 17.2879) (-55.9343, 17.239) (-55.9649, 17.1899) (-55.9952, 17.1408) (-56.0251, 17.0916) (-56.0548, 17.0423) (-56.084, 16.9929) (-56.1129, 16.9435) (-56.1415, 16.8939) (-56.1697, 16.8443) (-56.1975, 16.7946) (-56.225, 16.7448) (-56.2521, 16.695) (-56.2789, 16.6451) (-56.3053, 16.5951) (-56.3313, 16.545) (-56.3569, 16.4949) (-56.3822, 16.4447) (-56.4071, 16.3944) (-56.4316, 16.3441) (-56.4557, 16.2937) (-56.4794, 16.2433) (-56.5028, 16.1928) (-56.5258, 16.1422) (-56.5483, 16.0916) (-56.5705, 16.0409) (-56.5922, 15.9902) (-56.6136, 15.9394) (-56.6345, 15.8886) (-56.655, 15.8377) (-56.6751, 15.7868) (-56.6948, 15.7358) (-56.7141, 15.6848) (-56.7329, 15.6338) (-56.7513, 15.5827) (-56.7693, 15.5316) (-56.7868, 15.4805) (-56.8038, 15.4293) (-56.8204, 15.3781) (-56.8365, 15.3269) (-56.8521, 15.2757) (-56.8673, 15.2244) (-56.882, 15.1731) (-56.8963, 15.1218) (-56.91, 15.0705) (-56.9232, 15.0191) (-56.9358, 14.9678) (-56.9479, 14.9164) (-56.9594, 14.8651) (-56.9703, 14.8137) (-56.9808, 14.7624) (-56.9908, 14.7111) (-57.0003, 14.6597) (-57.0092, 14.6084) (-57.0173, 14.5571) (-57.0247, 14.5058) (-57.0311, 14.4546) (-57.0367, 14.4034) (-57.0415, 14.3522) (-57.0457, 14.3011) (-57.0495, 14.2501) (-57.0528, 14.199) (-57.0556, 14.1481) (-57.0572, 14.0972) (-57.0571, 14.0465) (-57.055, 14.0061) (-57.052, 13.9759) (-57.0494, 13.9559) (-57.0479, 13.9458) knots -1 -1 -1 -1 -1 -1 -0.98571429 -0.97142857 -0.95714286 -0.94285714 -0.92857143 -0.91428571 -0.9 -0.88571429 -0.87142857 -0.85714286 -0.84285714 -0.82857143 -0.81428571 -0.8 -0.78571429 -0.77142857 -0.75714286 -0.74285714 -0.72857143 -0.71428571 -0.7 -0.68571429 -0.67142857 -0.65714286 -0.64285714 -0.62857143 -0.61428571 -0.6 -0.58571429 -0.57142857 -0.55714286 -0.54285714 -0.52857143 -0.51428571 -0.5 -0.48571429 -0.47142857 -0.45714286 -0.44285714 -0.42857143 -0.41428571 -0.4 -0.38571429 -0.37142857 -0.35714286 -0.34285714 -0.32857143 -0.31428571 -0.3 -0.28571429 -0.27142857 -0.25714286 -0.24285714 -0.22857143 -0.21428571 -0.2 -0.18571429 -0.17142857 -0.15714286 -0.14285714 -0.12857143 -0.11428571 -0.1 -0.08571429 -0.07142857 -0.05714286 -0.04285714 -0.02857143 -0.01428571 0 0 0 0 0 0
  line L19 (-57.0479, 13.9458) -> (-56.8988, 12.9306)